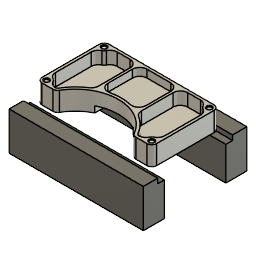
2D Adaptive Milling Tutorial (Autodesk Fusion 360 design; units mm, degrees)
Autodesk Fusion 360 part; units mm, degrees
sketch "Sketch1" plane through (0, 0, 0) normal (0, 1, 0) x (1, 0, 0)
  line L0 (75.946, 0) -> (75.946, 44.45)
  line L1 (75.946, 44.45) -> (0, 44.45)
  line L2 (0, 44.45) -> (0, 0)
  arc A0 (63.5707, 0) -> (12.3753, 0) centre (37.973, -12.7) ccw
  line L3 (0, 0) -> (12.3753, 0)
  line L4 (63.5707, 0) -> (75.946, 0)
  dimension "d1" = 75.946
  dimension "d2" = 44.45
  dimension "d3" = 12.7
  dimension "d4" = 28.575
  dimension "d5" = 37.973
  constraint horizontal L3
  constraint vertical L0
  constraint horizontal L1
  constraint vertical L2
  constraint coincident L2.end L3.start
  constraint collinear L3 L4
  measures "d1" distance of L2.end L0.start
  measures "d2" distance of L2.end L1.end
  measures "d3" vertical distance of L2.end A0.centre
  measures "d4" radius of A0
  measures "d5" distance of L2.end A0.centre L0.start
extrude "Extrude1" add sketch "Sketch1" against normal blind 12.7 makes body 1
fillet "Fillet1" radius 3.175 6 edges at (0, -6.35, 0) (12.3753, -6.35, 0) (63.5707, -6.35, 0) (75.946, -6.35, 0) (75.946, -6.35, -44.45) (0, -6.35, -44.45) on bodies 1
sketch "Sketch2" plane through (0, 0, 0) normal (0, 1, 0) x (-1, 0, 0)
  arc A0 (-3.175, -44.45) -> (0, -41.275) centre (-3.175, -41.275) ccw
  line L0 (0, -41.275) -> (0, -3.175)
  arc A1 (0, -3.175) -> (-3.175, 0) centre (-3.175, -3.175) ccw
  line L1 (-3.175, 0) -> (-10.4767, 0)
  arc A2 (-10.4767, 0) -> (-13.2263, -1.5875) centre (-10.4767, -3.175) ccw
  arc A3 (-62.7197, -1.5875) -> (-13.2263, -1.5875) centre (-37.973, 12.7) ccw
  arc A4 (-62.7197, -1.5875) -> (-65.4693, 0) centre (-65.4693, -3.175) ccw
  line L2 (-65.4693, 0) -> (-72.771, 0)
  arc A5 (-72.771, 0) -> (-75.946, -3.175) centre (-72.771, -3.175) ccw
  line L3 (-75.946, -3.175) -> (-75.946, -41.275)
  arc A6 (-75.946, -41.275) -> (-72.771, -44.45) centre (-72.771, -41.275) ccw
  line L4 (-72.771, -44.45) -> (-3.175, -44.45)
  line L5 (-1.778, -41.275) -> (-1.778, -3.175)
  arc A7 (-1.778, -3.175) -> (-3.175, -1.778) centre (-3.175, -3.175) ccw
  line L6 (-3.175, -1.778) -> (-10.4767, -1.778)
  arc A8 (-10.4767, -1.778) -> (-11.6865, -2.4765) centre (-10.4767, -3.175) ccw
  arc A9 (-64.2595, -2.4765) -> (-11.6865, -2.4765) centre (-37.973, 12.7) ccw
  arc A10 (-64.2595, -2.4765) -> (-65.4693, -1.778) centre (-65.4693, -3.175) ccw
  line L7 (-65.4693, -1.778) -> (-72.771, -1.778)
  arc A11 (-72.771, -1.778) -> (-74.168, -3.175) centre (-72.771, -3.175) ccw
  line L8 (-74.168, -3.175) -> (-74.168, -41.275)
  arc A12 (-74.168, -41.275) -> (-72.771, -42.672) centre (-72.771, -41.275) ccw
  line L9 (-72.771, -42.672) -> (-3.175, -42.672)
  arc A13 (-3.175, -42.672) -> (-1.778, -41.275) centre (-3.175, -41.275) ccw
  line L10 (-37.973, -44.45) -> (-37.973, -6.9842) construction
  line L11 (-25.273, -47.7039) -> (-25.273, -6.2054)
  line L12 (-23.749, -47.7039) -> (-23.749, -6.2054)
  line L13 (-50.673, -47.7039) -> (-50.673, -6.2054)
  line L14 (-52.197, -47.7039) -> (-52.197, -6.2054)
  arc A14 (0, -41.275) -> (-3.175, -44.45) centre (-3.175, -41.275) ccw
  arc A15 (-72.771, -44.45) -> (-75.946, -41.275) centre (-72.771, -41.275) ccw
  arc A16 (-75.946, -3.175) -> (-72.771, 0) centre (-72.771, -3.175) ccw
  arc A17 (-3.175, 0) -> (0, -3.175) centre (-3.175, -3.175) ccw
  dimension "d9" = -1.778
  dimension "d10" = 1.524
  dimension "d11" = 12.7
  constraint midpoint L4 L10.start
  constraint perpendicular L9 L10
  constraint vertical L11
  constraint symmetric L10 L11.start L13.start
  constraint symmetric L10 L11.end L13.end
  constraint symmetric L10 L12.start L14.start
  constraint symmetric L10 L12.end L14.end
  constraint coincident A0.start L4.end
  constraint coincident A0.centre A13.centre
  constraint coincident A6.end L4.start
  constraint coincident L3.end A6.start
  constraint coincident L2.end A5.start
  constraint coincident A5.end L3.start
  constraint coincident L0.end A1.start
  constraint coincident A1.end L1.start
  measures "d11" distance of L10 L11
extrude "Extrude2" cut sketch "Sketch2" against normal blind 8.255 contours L5 L6 A8 A9 L9 L12 A14 A17 | A9 A10 L7 L8 L9 L14 A15 A16 bodies 1
extrude "Extrude3" cut sketch "Sketch2" against normal blind 5.08 contours A9 L9 L11 L13 bodies 1
fillet "Fillet2" radius 4.826 16 edges at (6.0261, -4.1275, -42.672) (1.778, -4.1275, -38.4239) (1.778, -4.1275, -6.0261) (6.0261, -4.1275, -1.778) (23.749, -4.1275, -14.1138) (23.749, -4.1275, -42.672) (50.673, -2.54, -42.672) (69.9199, -4.1275, -42.672) (74.168, -4.1275, -38.4239) (25.273, -2.54, -42.672) (25.273, -2.54, -14.8684) (50.673, -2.54, -14.8684) (69.9199, -4.1275, -1.778) (74.168, -4.1275, -6.0261) (52.197, -4.1275, -42.672) (52.197, -4.1275, -14.1138) on bodies 1
hole "Hole1" at (3.175, 0, -41.275) at (3.175, 0, -3.175) at (72.771, 0, -3.175) at (72.771, 0, -41.275) direction (0, -1, 0) diameter 2.7686 depth 9.144 tip angle 118 countersink diameter 3.683 countersink angle 90 bodies 1
thread "Thread1" "ANSI Unified Screw Threads 0.138(#6) 6-32 UNC 2B" thread offset 0 thread depth 6.096
sketch "Sketch3" plane through (0, -12.7, 0) normal (0, -1, 0) x (1, 0, 0)
  arc A0 (0, -41.275) -> (3.175, -44.45) centre (3.175, -41.275) ccw
  line L0 (3.175, -44.45) -> (72.771, -44.45)
  arc A1 (72.771, -44.45) -> (75.946, -41.275) centre (72.771, -41.275) ccw
  line L1 (75.946, -41.275) -> (75.946, -3.175)
  arc A2 (75.946, -3.175) -> (72.771, 0) centre (72.771, -3.175) ccw
  line L2 (72.771, 0) -> (65.4693, 0)
  arc A3 (65.4693, 0) -> (62.7197, -1.5875) centre (65.4693, -3.175) ccw
  arc A4 (13.2263, -1.5875) -> (62.7197, -1.5875) centre (37.973, 12.7) ccw
  arc A5 (13.2263, -1.5875) -> (10.4767, 0) centre (10.4767, -3.175) ccw
  line L3 (10.4767, 0) -> (3.175, 0)
  arc A6 (3.175, 0) -> (0, -3.175) centre (3.175, -3.175) ccw
  line L4 (0, -3.175) -> (0, -41.275)
  line L5 (37.973, -44.45) -> (37.973, -7.62)
  line L6 (50.673, -9.525) -> (25.273, -9.525)
  line L7 (25.273, -9.525) -> (25.273, -42.545)
  line L8 (25.273, -42.545) -> (50.673, -42.545)
  line L9 (50.673, -42.545) -> (50.673, -9.525)
  line L10 (50.673, -9.525) -> (25.273, -42.545) construction
  line L11 (25.273, -9.525) -> (50.673, -42.545) construction
  point P0 (37.973, -26.035)
  dimension "d24" = 33.02
  dimension "d25" = 25.4
  constraint midpoint L0 L5.start
  constraint perpendicular L0 L5
  constraint perpendicular L6 L7
  constraint parallel L6 L8
  constraint parallel L7 L9
  constraint horizontal L6
  constraint coincident L10 P0
  constraint coincident L11 P0
  constraint midpoint L5 P0
  measures "d24" distance of L6.end L7.end
  measures "d25" distance of L7.end L8.end
extrude "Extrude4" cut sketch "Sketch3" against normal blind 4.191 contours A4 L5 L7 L8 | A4 L5 L8 L9 bodies 1
fillet "Fillet3" radius 8.128 2 edges at (50.673, -10.6045, -42.545) (25.273, -10.6045, -42.545) on bodies 1
ref_plane "WorkPlane1" through (37.973, -6.35, -22.225) normal (1, 0, 0) x (0, 0, 1)
sketch "Sketch4" plane through (37.973, -6.35, -22.225) normal (1, 0, 0) x (0, 0, -1)
  line L0 (0, 0) -> (0, -17.7867)
  line L1 (-17.4102, -10.541) -> (14.5751, -10.541)
  line L2 (19.05, -6.35) -> (-19.05, -6.35)
  line L3 (20.32, -10.541) -> (34.29, -10.541)
  line L4 (34.29, -10.541) -> (34.29, -32.766)
  line L5 (34.29, -32.766) -> (20.32, -32.766)
  line L6 (20.32, -32.766) -> (20.32, -10.541)
  line L7 (34.29, -10.541) -> (24.765, -10.541)
  line L8 (24.765, -10.541) -> (24.765, -7.366)
  line L9 (24.765, -7.366) -> (34.29, -7.366)
  line L10 (34.29, -7.366) -> (34.29, -10.541)
  line L11 (-34.29, -10.541) -> (-24.765, -10.541)
  line L12 (-34.29, -7.366) -> (-34.29, -10.541)
  line L13 (-24.765, -7.366) -> (-34.29, -7.366)
  line L14 (-20.32, -32.766) -> (-20.32, -10.541)
  line L15 (-24.765, -10.541) -> (-24.765, -7.366)
  line L16 (-20.32, -10.541) -> (-34.29, -10.541)
  line L17 (-34.29, -32.766) -> (-20.32, -32.766)
  line L18 (-34.29, -10.541) -> (-34.29, -32.766)
  dimension "d29" = 4.191
  dimension "d30" = 22.225
  dimension "d31" = 13.97
  dimension "d32" = 3.175
  dimension "d33" = 9.525
  dimension "d34" = 20.32
  constraint vertical L0
  constraint perpendicular L0 L1
  constraint horizontal L3
  constraint vertical L4
  constraint horizontal L5
  constraint vertical L6
  constraint horizontal L7
  constraint vertical L8
  constraint horizontal L9
  constraint vertical L10
  constraint coincident L0.start origin
  constraint symmetric L0 L3.start L14.end
  constraint symmetric L0 L3.end L11.start
  constraint symmetric L0 L4.end L17.start
  constraint symmetric L0 L5.end L14.start
  constraint symmetric L0 L7.end L11.end
  constraint symmetric L0 L8.end L13.start
  constraint symmetric L0 L9.end L12.start
  measures "d29" distance of L1 L2
  measures "d30" distance of L3.end L4.end
  measures "d31" distance of L3.start L3.end
  measures "d32" distance of L3.end L9.end
  measures "d33" distance of L8.end L9.end
  measures "d34" distance of L0 L6
extrude "Extrude5" add sketch "Sketch4" along normal mid plane 88.9 separate body makes body 2 at (23.1563, -22.1827, 12.065) makes body 3 at (52.7897, -30.6493, -56.515)
